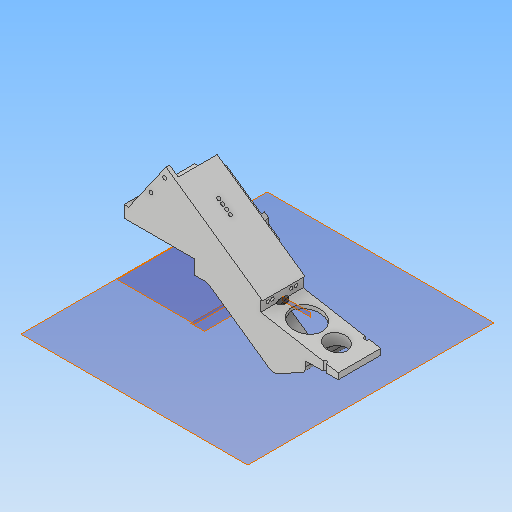
# Autodesk Inventor part: cellSTORM_inverted_opticsmodule_v0
Saved by Autodesk Inventor 2019.4 (Build 234330000, 330)
## iProperties
Created: 2020-11-06
Part Number: cellSTORM_inverted_opticsmodule_v0
Material: Generic
Document SubType Name: Modeling
Designer: diederichbenedict
Density: 1 g/cm^3
Appearance: Default
Author: diederichbenedict
Autodesk Inventor part; units mm, degrees
ref_plane "Work Plane3" through (-115.9521, -96.7438, -58.2763) normal (0, 0, -1) x (1, 0, 0)
sketch "Sketch1" plane through (-115.9521, -96.7438, -58.2763) normal (0, 0, -1) x (1, 0, 0)
  line L0 (-7, 0.25) -> (36, 0.25) construction
  line L1 (-7, 0.25) -> (-7, -8.45) construction
  line L2 (-7, -8.45) -> (-4, -8.45) construction
  line L3 (-4, -8.45) -> (-4, -14.75) construction
  line L4 (-1, -14.25) -> (-1, -7.5) construction
  line L5 (1, -17.25) -> (1, -14.75) construction
  line L6 (29, -17.25) -> (1, -17.25) construction
  line L7 (29, -14.75) -> (29, -17.25) construction
  line L8 (31, -14.75) -> (29, -14.75) construction
  line L9 (31, -17.25) -> (31, -14.75) construction
  line L10 (36, -17.25) -> (31, -17.25) construction
  line L11 (36, 0.25) -> (36, -17.25) construction
  line L12 (1, -7.5) -> (-1, -7.5) construction
  line L13 (1, -10) -> (1, -7.5) construction
  line L14 (29, -10) -> (1, -10) construction
  line L15 (29, -7.5) -> (29, -10) construction
  line L16 (31, -7.5) -> (29, -7.5) construction
  line L17 (31, -14.25) -> (31, -7.5) construction
  line L18 (-1, -14.25) -> (31, -14.25) construction
  line L19 (1, -0.25) -> (-1, -0.25) construction
  line L20 (1, -2.75) -> (1, -0.25) construction
  line L21 (29, -2.75) -> (1, -2.75) construction
  line L22 (29, -0.25) -> (29, -2.75) construction
  line L23 (31, -0.25) -> (29, -0.25) construction
  line L24 (31, -7) -> (31, -0.25) construction
  line L25 (-1, -7) -> (31, -7) construction
  line L26 (27.7903, 26.3233) -> (5.7037, 37.8208) construction
  line L27 (2.8269, 32.836) -> (5.3665, 37.7145) construction
  line L28 (25.357, 21.1075) -> (27.8966, 25.9861) construction
  line L29 (-43.6987, 4.97) -> (-31.4491, 13.5472) construction
  line L30 (-26.2161, -19.9978) -> (-13.9665, -11.4205) construction
  line L31 (-59.0209, -41.7593) -> (-53.082, -37.6009) construction
  line L32 (-75.3678, -18.4135) -> (-69.429, -14.2551) construction
  line L33 (-83.9784, -25.1198) -> (-79.8757, -30.9791) construction
  line L34 (31, 7.25) -> (31, 25.7798)
  line L35 (31, 25.7798) -> (3.201, 40.2511)
  line L36 (-100.2578, -32.1915) -> (-80.1961, -60.8425)
  line L37 (-80.1961, -60.8425) -> (-5.6575, -8.65)
  line L38 (-5.6575, -8.65) -> (-7.2, -8.65)
  line L39 (-7.2, -8.65) -> (-7.2, 0.45)
  line L40 (10.553, 27.4048) -> (-77.5642, -34.2955) construction
  line L41 (-7.2, 0.45) -> (31, 7.25)
  line L42 (-69.0481, -49.0348) -> (-79.0921, -56.3322) construction
  line L43 (-95.9265, -32.2901) -> (-85.6341, -25.3477) construction
  line L44 (-63.1835, 5.33) -> (-63.1835, -10.67) construction
  line L45 (-63.1835, -10.67) -> (-65.1835, -10.67) construction
  line L46 (-69.5218, -10.67) -> (-63.1835, -10.67)
  line L47 (-63.1835, -10.67) -> (-63.1835, -6.2318)
  line L48 (3.201, 40.2511) -> (-63.1835, -6.2318)
  line L49 (-69.5218, -10.67) -> (-100.2578, -32.1915)
  line L50 (1, -14.75) -> (-4, -14.75) projected
  line L51 (-1, -7) -> (-1, -0.25) projected
  point P0 (115.9521, -96.7438)
  point P1 (-1, -14.75)
  dimension "d1" = 1
  dimension "d3" = 0.2
  dimension "d4" = 0.2
  dimension "d6" = 0
  dimension "d7" = 0.2
  dimension "d8" = 7
  dimension "d9" = 3
  dimension "d92" = 0
  dimension "d114" = 95
  constraints: 34 end point, 3 perpendicular, 2 horizontal, 2 parallel, 1 point on line, 1 vertical, 15 other
  measures "d1" distance between parallel lines of L26 L35
  measures "d3" distance between parallel lines of L2 L38
  measures "d4" distance between parallel lines of L1 L39
  measures "d6" distance between parallel lines of L34 L24
  measures "d7" distance from line of L39.end L0
  measures "d8" distance from line of L0 L34.start
  measures "d9" distance from line of L36.end L42
  measures "d92" angle of L48 L37
  measures "d114" distance from line of L36 L0.start
extrude "Extrusion1" add sketch "Sketch1" against normal blind 3
ref_plane "Work Plane4" through (-106.9756, -82.4938, -91.2763) normal (0, 0, 1) x (1, 0, 0)
sketch "Sketch2" plane through (-115.9521, -96.7438, -58.2763) normal (0, 0, -1) x (-1, 0, 0)
  line L0 (-31, -25.7798) -> (-31, -7.25)
  line L1 (-3.201, -40.2511) -> (-31, -25.7798)
  line L2 (63.1835, 6.2318) -> (-3.201, -40.2511)
  line L3 (80.1961, 60.8425) -> (100.2578, 32.1915)
  line L4 (5.6575, 8.65) -> (80.1961, 60.8425)
  line L5 (7.2, 8.65) -> (5.6575, 8.65)
  line L6 (7.2, -0.45) -> (7.2, 8.65)
  line L7 (-31, -7.25) -> (7.2, -0.45)
  line L8 (59.0209, 41.7593) -> (53.082, 37.6009) construction
  line L9 (75.3678, 18.4135) -> (69.429, 14.2551)
  line L10 (-3.2205, -36.8588) -> (-28, -23.9593)
  line L11 (-28, -23.9593) -> (-28, -9.7631)
  line L12 (-28, -9.7631) -> (10.2, -2.9631)
  line L13 (10.2, -2.9631) -> (10.2, 11.65) construction
  line L14 (71.0992, 15.4246) -> (54.7523, 38.7704)
  line L15 (59.0209, 41.7593) -> (53.082, 37.6009)
  line L16 (65.1603, 11.2662) -> (48.8134, 34.612) construction
  line L17 (75.3678, 18.4135) -> (69.429, 14.2551)
  line L18 (46.6751, 33.3589) -> (61.0457, 12.8355)
  line L19 (82.2228, 22.9692) -> (75.8066, 18.4766)
  line L20 (10.2, 7.8187) -> (46.6751, 33.3589)
  line L21 (10.2, 7.8187) -> (26.7764, -15.8547)
  line L22 (10.2, -2.9631) -> (21.7105, -19.4019)
  line L23 (80.1961, 60.8425) -> (100.2578, 32.1915)
  line L24 (100.2578, 32.1915) -> (-3.201, -40.2511)
  line L25 (63.1835, 10.67) -> (63.1835, 6.2318)
  line L26 (69.5218, 10.67) -> (63.1835, 10.67)
  line L27 (100.2578, 32.1915) -> (69.5218, 10.67)
  line L28 (60.1835, 7.5372) -> (60.1835, 12.2317)
  line L29 (60.1835, 12.2317) -> (61.0457, 12.8355)
  line L30 (63.1835, 10.67) -> (63.1835, 6.2318)
  line L31 (60.1835, 7.5372) -> (-3.2205, -36.8588)
  line L32 (63.1835, 6.2318) -> (-3.201, -40.2511)
  line L33 (63.1835, 10.67) -> (63.1835, 6.2318)
  line L34 (63.1835, 6.2318) -> (63.1835, 10.67)
  line L35 (100.2578, 32.1915) -> (69.5218, 10.67)
  line L36 (63.1835, 10.67) -> (69.5218, 10.67)
  line L37 (69.5218, 10.67) -> (100.2578, 32.1915)
  line L38 (-28, -19.2299) -> (0.6537, -34.146)
  line L39 (75.3678, 18.4135) -> (59.0209, 41.7593) construction
  line L40 (59.0209, 41.7593) -> (53.082, 37.6009) construction
  line L41 (69.429, 14.2551) -> (53.082, 37.6009) construction
  line L42 (75.3678, 18.4135) -> (69.429, 14.2551) construction
  line L43 (75.3678, 18.4135) -> (59.0209, 41.7593) construction
  line L44 (59.0209, 41.7593) -> (53.082, 37.6009) construction
  line L45 (69.429, 14.2551) -> (53.082, 37.6009) construction
  line L46 (75.3678, 18.4135) -> (69.429, 14.2551) construction
  line L47 (75.3678, 18.4135) -> (59.0209, 41.7593) construction
  line L48 (59.0209, 41.7593) -> (53.082, 37.6009) construction
  line L49 (69.429, 14.2551) -> (53.082, 37.6009) construction
  line L50 (75.3678, 18.4135) -> (69.429, 14.2551) construction
  line L51 (69.429, 14.2551) -> (53.082, 37.6009) construction
  line L52 (75.3678, 18.4135) -> (69.429, 14.2551) construction
  line L53 (49.2033, 35.1291) -> (79.6237, 56.4297)
  line L54 (79.6237, 56.4297) -> (96.2, 32.7562)
  line L55 (96.2, 32.7562) -> (66.1366, 11.7056)
  line L56 (49.2033, 35.1291) -> (66.1366, 11.7056)
  line L57 (65.2751, 11.1023) -> (65.1603, 11.2662)
  line L58 (63.1835, 14.0894) -> (63.0694, 14.2524)
  line L59 (48.8134, 34.612) -> (48.6987, 34.7758)
  point P0 (-115.9521, 96.7438)
extrude "Extrusion2" add sketch "Sketch2" along normal up to surface (33 mm away) contours L0 L7 L6 L5 L4 L3 L24 L26 L25 L2 L1
sketch "Sketch3" plane through (-112.7316, -133.6026, -58.2763) normal (-0.4617486, 0.8870108, 0) x (0.8870108, 0.4617486, 0)
  circle A0 centre (14.2084, 15) radius 12.7 projected
  line L0 (0, 33) -> (27.936, 33) projected
  line L1 (0, 0) -> (0, 33) projected
  line L2 (27.936, 0) -> (0, 0) projected
  line L3 (27.936, 0) -> (27.936, 33) projected
  circle A1 centre (14.2084, 15) radius 13.2
  point P0 (161.685, -58.2763)
  dimension "d15" = 0.5
  constraints: 1 centre point
  measures "d15" radial gap between concentric circles of A0 A1
ref_plane "Work Plane5" through (-110.6706, -134.7844, -86.2023) normal (0.4617486, -0.8870108, 0) x (0.8863364, 0.4613975, -0.0389899)
extrude "Extrusion3" cut sketch "Sketch3" against normal blind 2.2 contours A0 | A1
sketch "Sketch4" plane through (-99.1128, -128.9933, -73.2763) normal (-0.4617486, 0.8870108, 0) x (0.8870108, 0.4617486, 0)
  circle A0 centre (0, 0) radius 13.2 projected
  circle A1 centre (0, 0) radius 8.2
  point P0 (147.4766, -73.2763)
  dimension "d18" = 5
  constraints: 1 centre point
  measures "d18" radial gap between concentric circles of A0 A1
extrude "Extrusion4" cut sketch "Sketch4" against normal blind 3 contours A1
ref_plane "Work Plane6" through (-115.6592, -109.4938, -86.9599) normal (0, 1, 0) x (0.2856174, 0, 0.9583437)
sketch "Sketch5" plane through (-128.1477, 0, -58.2763) normal (0, 1, 0) x (1, 0, 0)
  circle A0 centre (26.1721, 15) radius 12.15 projected
  circle A1 centre (26.1721, 15) radius 13
  point P0 (128.1477, -58.2763)
  point P1 (24.1765, 18)
  dimension "d145" = 26
  constraints: 1 centre point, 1 coincident
  measures "d145" diameter of A1
extrude "Extrusion5" cut sketch "Sketch5" against normal up to surface (109.4938 mm away) contours A0 | A1
sketch "Sketch6" plane through (-216.2099, -64.5523, -91.2763) normal (-0.819152, 0.5735764, 0) x (0, 0, 1)
  circle A0 centre (18, 17.24) radius 12.3
  circle A1 centre (18, 17.24) radius 14.6
  point P0 (91.2763, 176.891)
  dimension "d113" = 29.2
  constraints: 2 centre point, 2 other
  measures "d113" diameter of A1
extrude "Extrusion6" cut sketch "Sketch6" against normal up to surface (3 mm away) contours A0 | A1
sketch "Sketch10" plane through (-84.9521, -122.5236, -91.2763) normal (0, 0, -1) x (-1, 0, 0)
  line L0 (38.2, 25.3298) -> (0, 18.5298) construction
  line L1 (0, 18.5298) -> (0, 0) construction
  line L2 (0, 0) -> (27.799, -14.4713) construction
  line L3 (27.799, -14.4713) -> (94.1835, 32.0116) construction
  line L4 (131.2578, 57.9713) -> (111.1961, 86.6223) construction
  line L5 (111.1961, 86.6223) -> (36.6575, 34.4298) construction
  line L6 (36.6575, 34.4298) -> (38.2, 34.4298) construction
  line L7 (38.2, 34.4298) -> (38.2, 25.3298) construction
  line L8 (3, 1.8204) -> (3, 16.0167) construction
  line L9 (3, 16.0167) -> (41.2, 22.8167) construction
  line L10 (41.2, 22.8167) -> (52.7105, 6.3779) construction
  line L11 (27.7795, -11.079) -> (3, 1.8204) construction
  line L12 (96.1835, 36.4498) -> (152.1835, 36.4498) construction
  line L13 (94.1835, 20.4498) -> (94.1835, 36.4498) construction
  line L14 (154.1835, 20.4498) -> (154.1835, 36.4498) construction
  line L15 (100.5218, 36.4498) -> (154.1835, 36.4498) construction
  line L16 (100.5218, 36.4498) -> (154.1835, 36.4498) construction
  line L17 (131.2578, 57.9713) -> (27.799, -14.4713) construction
  line L18 (154.1835, 46.4498) -> (154.1835, 36.4498)
  line L19 (111.1961, 86.6223) -> (131.2578, 57.9713) construction
  line L20 (131.2578, 57.9713) -> (100.5218, 36.4498) construction
  line L21 (94.1835, 32.0116) -> (94.1835, 24.4498) construction
  line L22 (94.1835, 24.4498) -> (83.3841, 24.4498)
  line L23 (94.1835, 32.0116) -> (83.3841, 24.4498) construction
  line L24 (154.1835, 36.4498) -> (100.5218, 36.4498)
  line L25 (131.2578, 57.9713) -> (100.5218, 36.4498)
  line L26 (83.3841, 24.4498) -> (94.1835, 32.0116)
  line L27 (94.1835, 24.4498) -> (94.1835, 32.0116)
  line L28 (94.1835, 36.4498) -> (100.5218, 36.4498) projected
  line L29 (100.5218, 36.4498) -> (131.2578, 57.9713) projected
  line L30 (94.1835, 32.0116) -> (94.1835, 36.4498) projected
  line L31 (91.1835, 33.317) -> (57.7764, 9.925) projected
  line L32 (52.7105, 6.3779) -> (27.7795, -11.079) projected
  line L33 (57.7764, 9.925) -> (41.2, 33.5985) projected
  line L34 (41.2, 33.5985) -> (77.6751, 59.1387) projected
  line L35 (77.6751, 59.1387) -> (92.0457, 38.6153) projected
  line L36 (92.0457, 38.6153) -> (91.1835, 38.0115) projected
  line L37 (91.1835, 38.0115) -> (91.1835, 33.317) projected
  line L38 (83.3841, 24.4498) -> (81.7838, 26.7352)
  line L39 (127.2, 58.536) -> (97.1366, 37.4854) construction
  line L40 (57.7764, 9.925) -> (91.1835, 33.317) projected
  line L41 (81.7838, 26.7352) -> (91.1835, 33.317)
  line L42 (91.1835, 33.317) -> (91.1835, 38.0115) projected
  line L43 (91.1835, 33.317) -> (91.1835, 38.0115)
  line L44 (91.1835, 38.0115) -> (92.0457, 38.6153) construction
  line L45 (92.0457, 38.6153) -> (94.9309, 40.6355)
  line L46 (94.9309, 40.6355) -> (97.1366, 37.4854) construction
  line L47 (97.1366, 37.4854) -> (127.2, 58.536) construction
  line L48 (94.9309, 40.6355) -> (97.1366, 37.4854)
  line L49 (97.1366, 37.4854) -> (127.2, 58.536)
  line L50 (127.2, 58.536) -> (130.8624, 58.536)
  line L51 (100.5218, 36.4498) -> (131.2578, 57.9713) projected
  line L52 (130.8624, 58.536) -> (131.2578, 57.9713)
  line L53 (57.7764, 9.925) -> (91.1835, 33.317) projected
  line L54 (81.7838, 26.7352) -> (91.1835, 33.317)
  line L55 (91.1835, 33.317) -> (91.1835, 38.0115)
  line L56 (91.1835, 38.0115) -> (94.9309, 40.6355)
  line L57 (94.9309, 40.6355) -> (97.1366, 37.4854)
  line L58 (154.1835, 46.4498) -> (114.8033, 46.4498)
  line L59 (131.2578, 57.9713) -> (100.5218, 36.4498) projected
  point P0 (-84.9521, 122.5236)
  dimension "d38" = 12
  dimension "d149" = 10
  constraints: 50 end point, 13 point on line, 11 collinear, 7 perpendicular, 2 horizontal, 2 vertical, 1 parallel
  measures "d38" distance between parallel lines of L12 L22
  measures "d149" distance between parallel lines of L58 L12
ref_plane "Work Plane7" through (-237.1356, -102.0738, -103.2763) normal (0, 0, -1) x (0, 1, 0)
extrude "Extrusion10" add sketch "Sketch10" against normal blind 36 and the other way blind 24 contours L18 L24 L25 L58 | L27 L22 L26
sketch "Sketch11" plane through (-84.9521, -122.5236, -91.2763) normal (0, 0, -1) x (-1, 0, 0)
  line L0 (57.7764, 9.925) -> (91.1835, 33.317) projected
  line L1 (58.8799, 51.3735) -> (38, 37.4298) projected
  circle A0 centre (58.4518, 12.1681) radius 1.45
  line L2 (41.7774, 33.4536) -> (57.8377, 10.5172) projected
  line L3 (52.7105, 6.3779) -> (27.7795, -11.079) projected
  arc A1 (61.4816, 12.5195) -> (55.7249, 13.5345) centre (58.4518, 12.1681) ccw
  line L4 (91.1835, 33.317) -> (57.7764, 9.925) projected
  line L5 (38.2, 25.3298) -> (0, 18.5298) projected
  line L6 (0, 18.5298) -> (0, 0) projected
  line L7 (0, 0) -> (27.799, -14.4713) projected
  line L8 (27.799, -14.4713) -> (83.3841, 24.4498) projected
  line L9 (83.3841, 24.4498) -> (94.1835, 32.0116) projected
  line L10 (94.1835, 32.0116) -> (94.1835, 36.4498) projected
  line L11 (94.1835, 36.4498) -> (100.5218, 36.4498) projected
  line L12 (131.2578, 57.9713) -> (111.1961, 86.6223) projected
  line L13 (111.1961, 86.6223) -> (36.6575, 34.4298) projected
  line L14 (36.6575, 34.4298) -> (38.2, 34.4298) projected
  line L15 (38.2, 34.4298) -> (38.2, 25.3298) projected
  line L16 (3, 1.8204) -> (3, 16.0167) projected
  line L17 (3, 16.0167) -> (41.2, 22.8167) projected
  line L18 (41.2, 22.8167) -> (52.7105, 6.3779) projected
  line L19 (27.7795, -11.079) -> (3, 1.8204) projected
  circle A2 centre (50.6911, 6.734) radius 1.45
  line L20 (41.2, 22.8167) -> (52.7105, 6.3779) projected
  line L21 (52.7105, 6.3779) -> (27.7795, -11.079) projected
  line L22 (52.7105, 6.3779) -> (41.2, 22.8167) projected
  arc A3 (50.6911, 9.262) -> (49.8265, 4.3585) centre (50.6911, 6.734) ccw
  circle A4 centre (43.9558, 33.2951) radius 1.45
  circle A5 centre (43.9558, 33.2951) radius 3.503
  line L23 (41.2, 33.5985) -> (57.7764, 9.925) projected
  line L24 (41.2, 22.8167) -> (3, 16.0167) projected
  line L25 (3, 16.0167) -> (3, 1.8204) projected
  line L26 (3, 1.8204) -> (27.7795, -11.079) projected
  line L27 (52.7105, 6.3779) -> (41.2, 22.8167) projected
  line L28 (91.1835, 33.317) -> (91.1835, 38.0115) projected
  line L29 (91.1835, 38.0115) -> (92.0457, 38.6153) projected
  line L30 (92.0457, 38.6153) -> (77.6751, 59.1387) projected
  line L31 (77.6751, 59.1387) -> (41.2, 33.5985) projected
  line L32 (41.2, 33.5985) -> (57.7764, 9.925) projected
  line L33 (27.7795, -11.079) -> (52.7105, 6.3779) projected
  line L34 (52.7105, 6.3779) -> (27.7795, -11.079) projected
  line L35 (57.7764, 9.925) -> (41.2, 33.5985) projected
  line L36 (41.2, 33.5985) -> (77.6751, 59.1387) projected
  line L37 (77.6751, 59.1387) -> (92.0457, 38.6153) projected
  line L38 (92.0457, 38.6153) -> (91.1835, 38.0115) projected
  line L39 (91.1835, 38.0115) -> (91.1835, 33.317) projected
  line L40 (100.5218, 36.4498) -> (114.8033, 46.4498) projected
  line L41 (114.8033, 46.4498) -> (131.2578, 57.9713) projected
  point P0 (-84.9521, 122.5236)
  point P1 (61.747, 47.4364)
  point P2 (77.9448, 24.3035)
  point P3 (77.8072, 24.5)
  point P4 (43.8644, 29.7933)
  point P5 (45.3538, 36.5071)
  point P6 (40.4594, 33.08)
  point P7 (40.5297, 32.5651)
  dimension "d44" = 2.9
  dimension "d47" = 2.9
  dimension "d96" = 2.9
  constraints: 8 point on circle, 6 centre point, 4 point on line, 4 tangent, 3 coincident, 2 other
  measures "d44" diameter of A0
  measures "d47" diameter of A2
  measures "d96" diameter of A4
extrude "Extrusion11" add sketch "Sketch11" against normal up to surface (36 mm away) contours A3 L18 A2 L3 | A2 L18 L3
fillet "Fillet1" radius 7 6 edges at (-112.7512, -136.9949, -73.2763) (-84.9521, -122.5236, -73.2763) (-168.3362, -98.0738, -73.2763) (-112.7316, -133.6026, -74.7763) (-87.9521, -120.7032, -74.7763) (-87.9521, -106.5069, -74.7763)
sketch "Sketch13" plane through (-123.1521, -88.0938, -55.2763) normal (1, 0, 0) x (0, 0, -1)
  circle A0 centre (10, -4.4426) radius 1.45 projected
  circle A1 centre (26, -4.4426) radius 1.45 projected
  circle A2 centre (30, -4.4426) radius 1.45 projected
  circle A3 centre (6, -4.4426) radius 1.45 projected
  point P0 (-55.2763, 88.0938)
extrude "Extrusion13" cut sketch "Sketch13" against normal blind 25
sketch "Sketch16" plane through (-163.179, -96.2524, -91.2763) normal (0, 0, -1) x (-1, 0, 0)
  line L0 (53.0309, 31.7002) -> (32.9692, 60.3512) projected
  line L1 (32.9692, 60.3512) -> (-41.5694, 8.1586) projected
  line L2 (-78.2269, -7.7414) -> (-40.0269, -0.9414) projected
  line L3 (-78.2269, -7.7414) -> (-105.7935, -12.6485)
  line L4 (-105.2267, -17.7414) -> (-97.798, -17.7414) projected
  line L5 (-105.7935, -12.6485) -> (-105.7935, -17.7414)
  line L6 (-105.7935, -17.7414) -> (-78.2269, -17.7414)
  line L7 (-78.2269, -22.0234) -> (-78.2269, -7.7414) projected
  line L8 (-78.2269, -7.7414) -> (-78.2269, -17.7414)
  line L9 (-41.5694, 8.1586) -> (-40.0269, 8.1586) projected
  line L10 (-40.0269, 8.1586) -> (-40.0269, -0.9414) projected
  line L11 (-40.0269, -0.9414) -> (-78.2269, -7.7414) projected
  line L12 (-78.2269, -7.7414) -> (-78.2269, -22.0234) projected
  arc A0 (-78.2269, -22.0234) -> (-74.4591, -28.2325) centre (-71.2269, -22.0234) ccw projected
  line L13 (-74.4591, -28.2325) -> (-54.1956, -38.781) projected
  arc A1 (-54.1956, -38.781) -> (-46.9483, -38.306) centre (-50.9634, -32.572) ccw projected
  line L14 (-46.9483, -38.306) -> (3.3492, -3.0873) projected
  arc A2 (7.3643, -1.8214) -> (3.3492, -3.0873) centre (7.3643, -8.8214) ccw projected
  line L15 (5.1572, -1.8214) -> (7.3643, -1.8214) projected
  line L16 (5.1572, -1.8214) -> (15.9566, 5.7405) projected
  line L17 (15.9566, 5.7405) -> (15.9566, 10.1786) projected
  line L18 (15.9566, 10.1786) -> (22.2949, 10.1786) projected
  line L19 (-20.4505, -16.3461) -> (-37.0269, 7.3274) projected
  line L20 (-37.0269, 7.3274) -> (-0.5518, 32.8675) projected
  line L21 (-0.5518, 32.8675) -> (13.8188, 12.3441) projected
  line L22 (13.8188, 12.3441) -> (12.9566, 11.7403) projected
  line L23 (12.9566, 11.7403) -> (12.9566, 7.0458) projected
  line L24 (12.9566, 7.0458) -> (-20.4505, -16.3461) projected
  circle A3 centre (-27.5358, -19.5372) radius 1.45 projected
  arc A4 (-27.5358, -17.0092) -> (-28.4005, -21.9127) centre (-27.5358, -19.5372) ccw projected
  line L25 (-28.4005, -21.9127) -> (-46.9679, -34.9137) projected
  arc A5 (-54.2151, -35.3887) -> (-46.9679, -34.9137) centre (-50.9829, -29.1797) ccw projected
  line L26 (-54.2151, -35.3887) -> (-71.4591, -26.4121) projected
  arc A6 (-75.2269, -20.203) -> (-71.4591, -26.4121) centre (-68.2269, -20.203) ccw projected
  line L27 (-75.2269, -20.203) -> (-75.2269, -16.1185) projected
  arc A7 (-69.4537, -9.2268) -> (-75.2269, -16.1185) centre (-68.2269, -16.1185) ccw projected
  line L28 (-69.4537, -9.2268) -> (-37.0269, -3.4545) projected
  line L29 (-37.0269, -3.4545) -> (-27.5358, -17.0092) projected
  line L30 (22.2949, 10.1786) -> (36.5764, 20.1786) projected
  line L31 (36.5764, 20.1786) -> (53.0309, 31.7002) projected
  point P0 (-163.179, 96.2524)
  point P1 (-45.8001, -1.9691)
  dimension "d69" = 28
  constraints: 8 end point, 1 collinear, 1 point on line, 1 vertical
  measures "d69" distance of L2.start L3.end
extrude "Extrusion16" add sketch "Sketch16" against normal up to surface (36 mm away) contours L7 L6 L4 L5 L3
sketch "Sketch17" plane through (-84.9521, -113.9938, -91.2763) normal (0, -1, 0) x (1, 0, 0)
  arc A0 (8.0711, 22.55) -> (8.0711, 13.45) centre (8.0711, 18) ccw projected
  circle A1 centre (16.0711, 0.5) radius 2.1 projected
  arc A2 (16.0711, 37.6) -> (16.0711, 33.4) centre (16.0711, 35.5) ccw projected
  circle A3 centre (16.0711, 0.5) radius 1.7427
  circle A4 centre (16.0711, 35.5) radius 1.45
  circle A5 centre (8.0711, 18) radius 9
  point P0 (84.9521, 91.2763)
  dimension "d72" = 2.9
  dimension "d73" = 18
  constraints: 3 centre point, 3 coincident
  measures "d72" diameter of A4
  measures "d73" diameter of A5
extrude "Extrusion17" cut sketch "Sketch17" against normal through all contours A3 | A4 | A5
sketch "Sketch19" plane through (-84.9521, -122.5236, -115.2763) normal (0, 0, -1) x (-1, 0, 0)
  line L0 (31.259, -8.6426) -> (49.8265, 4.3585) projected
  line L1 (-14.4017, 15.9661) -> (-14.4017, 8.5298) projected
  line L2 (-14.4017, 8.5298) -> (0, 8.5298) projected
  line L3 (0, 8.5298) -> (0, 4.2477) projected
  arc A0 (0, 4.2477) -> (3.7678, -1.9614) centre (7, 4.2477) ccw projected
  line L4 (3.7678, -1.9614) -> (24.0313, -12.5099) projected
  arc A1 (24.0313, -12.5099) -> (31.2786, -12.0349) centre (27.2635, -6.3008) ccw projected
  line L5 (31.2786, -12.0349) -> (81.5761, 23.1839) projected
  arc A2 (85.5912, 24.4498) -> (81.5761, 23.1839) centre (85.5912, 17.4498) ccw projected
  line L6 (83.3841, 24.4498) -> (85.5912, 24.4498) projected
  line L7 (83.3841, 24.4498) -> (94.1835, 32.0116) projected
  line L8 (94.1835, 32.0116) -> (94.1835, 36.4498) projected
  line L9 (94.1835, 36.4498) -> (100.5218, 36.4498) projected
  line L10 (131.2578, 57.9713) -> (111.1961, 86.6223) projected
  line L11 (111.1961, 86.6223) -> (36.6575, 34.4298) projected
  line L12 (36.6575, 34.4298) -> (38.2, 34.4298) projected
  line L13 (38.2, 34.4298) -> (38.2, 25.3298) projected
  line L14 (38.2, 25.3298) -> (-14.4017, 15.9661) projected
  circle A3 centre (50.6911, 6.734) radius 1.45 projected
  line L15 (77.6751, 59.1387) -> (92.0457, 38.6153) projected
  line L16 (92.0457, 38.6153) -> (91.1835, 38.0115) projected
  line L17 (91.1835, 38.0115) -> (91.1835, 33.317) projected
  line L18 (91.1835, 33.317) -> (57.7764, 9.925) projected
  line L19 (57.7764, 9.925) -> (41.2, 33.5985) projected
  line L20 (41.2, 33.5985) -> (77.6751, 59.1387) projected
  line L21 (49.8265, 4.3585) -> (31.259, -8.6426) projected
  arc A4 (24.0118, -9.1176) -> (31.259, -8.6426) centre (27.244, -2.9085) ccw projected
  line L22 (24.0118, -9.1176) -> (6.7678, -0.1409) projected
  arc A5 (3, 6.0681) -> (6.7678, -0.1409) centre (10, 6.0681) ccw projected
  line L23 (3, 6.0681) -> (3, 10.1527) projected
  arc A6 (8.7732, 17.0444) -> (3, 10.1527) centre (10, 10.1527) ccw projected
  line L24 (8.7732, 17.0444) -> (41.2, 22.8167) projected
  line L25 (41.2, 22.8167) -> (50.6911, 9.262) projected
  arc A7 (50.6911, 9.262) -> (49.8265, 4.3585) centre (50.6911, 6.734) ccw projected
  line L26 (57.7764, 9.925) -> (91.1835, 33.317) projected
  line L27 (83.3841, 24.4498) -> (94.1835, 32.0116) projected
  line L28 (83.3841, 24.4498) -> (81.7838, 26.7352)
  line L29 (81.7838, 26.7352) -> (91.1835, 33.317)
  line L30 (91.1835, 38.0115) -> (92.0457, 38.6153) projected
  line L31 (91.1835, 33.317) -> (91.1835, 38.0115)
  line L32 (91.1835, 33.317) -> (91.1835, 38.0115) projected
  line L33 (91.1835, 38.0115) -> (94.9309, 40.6355)
  line L34 (94.9309, 40.6355) -> (97.1366, 37.4854)
  line L35 (97.1366, 37.4854) -> (127.2, 58.536) projected
  line L36 (97.1366, 37.4854) -> (127.2, 58.536)
  line L37 (127.2, 58.536) -> (130.8624, 58.536)
  line L38 (111.1961, 86.6223) -> (131.2578, 57.9713) projected
  line L39 (130.8624, 58.536) -> (127.162, 55.1034)
  line L40 (127.162, 55.1034) -> (100.5218, 36.4498)
  line L41 (100.5218, 36.4498) -> (94.1835, 36.4498)
  line L42 (94.1835, 36.4498) -> (94.1835, 32.0116)
  line L43 (98.2792, 34.8795) -> (83.3841, 24.4498)
  line L44 (100.5218, 36.4498) -> (114.8033, 46.4498) projected
  line L45 (114.8033, 46.4498) -> (131.2578, 57.9713) projected
  point P0 (-84.9521, 122.5236)
  point P1 (107.1198, 75.0095)
  point P2 (94.1835, 24.4498)
  constraints: 24 end point, 4 point on line, 3 perpendicular, 1 collinear, 1 horizontal, 1 parallel, 1 vertical, 2 other
extrude "Extrusion19" add sketch "Sketch19" against normal up to surface (24 mm away) contours L39 L40 L9 L8 L7 L28 L18 L17 L16 L33 L34 L35 L37 | L10 L45 L39
ref_plane "Work Plane9" through (-239.1356, -131.0738, -115.2763) normal (0, -1, 0) x (1, 0, 0)
ref_plane "Work Plane10" through (-239.1356, -131.0738, -115.2763) normal (0, -1, 0) x (1, 0, 0)
sketch "Sketch23" plane through (-115.9521, -96.7438, -55.2763) normal (0, 0, 1) x (1, 0, 0)
  line L0 (-80.1961, 60.8425) -> (-100.2578, 32.1915) projected
  line L1 (-99.8624, 32.7562) -> (-80.1961, 60.8425) projected
  line L2 (-80.1961, 60.8425) -> (-87.5685, 66.0047)
  line L3 (-87.5685, 66.0047) -> (-119.3122, 20.67)
  line L4 (-119.3122, 20.67) -> (-119.3122, 20.67)
  line L5 (-123.1835, 20.67) -> (-83.8033, 20.67) projected
  line L6 (-119.3122, 20.67) -> (-83.8033, 20.67)
  line L7 (-83.8033, 20.67) -> (-100.2578, 32.1915)
  line L8 (-80.1961, 60.8425) -> (-100.2578, 32.1915)
  line L9 (-100.2578, 32.1915) -> (-83.8033, 20.67)
  line L10 (-83.8033, 20.67) -> (-119.3122, 20.67)
  line L11 (-83.8033, 20.67) -> (-123.1835, 20.67) projected
  circle A0 centre (-100.2756, 41.0424) radius 1.6 projected
  circle A1 centre (-88.8041, 57.4255) radius 1.6 projected
  point P0 (115.9521, 96.7438)
  point P1 (-96.162, 29.3237)
  dimension "d146" = 9
  constraints: 16 end point, 3 collinear, 2 perpendicular, 2 point on line, 1 horizontal, 1 vertical, 1 other
extrude "Extrusion22" add sketch "Sketch23" against normal blind 3
sketch "Sketch24" plane through (-123.1521, -97.1938, -91.2763) normal (0, 0, -1) x (-1, 0, 0)
  line L0 (52.8428, 8.1328) -> (36.4959, 31.4786) construction
  line L1 (36.4959, 31.4786) -> (30.557, 27.3202) construction
  line L2 (46.9039, 3.9744) -> (30.557, 27.3202) construction
  line L3 (52.8428, 8.1328) -> (46.9039, 3.9744) construction
  line L4 (42.6395, 35.7805) -> (58.9864, 12.4346) construction
  line L5 (58.9864, 12.4346) -> (64.9253, 16.5931) construction
  line L6 (48.5783, 39.9389) -> (64.9253, 16.5931) construction
  line L7 (42.6395, 35.7805) -> (48.5783, 39.9389) construction
  circle A0 centre (12.4911, -18.5958) radius 1.45 construction
  line L8 (89, 33.2062) -> (92.6624, 33.2062) construction
  line L9 (92.6624, 33.2062) -> (72.9961, 61.2925) construction
  line L10 (72.9961, 61.2925) -> (-1.5425, 9.1) construction
  line L11 (-1.5425, 9.1) -> (0, 9.1) construction
  line L12 (0, 9.1) -> (0, 0) construction
  line L13 (0, 0) -> (-52.6017, -9.3636) construction
  line L14 (-52.6017, -9.3636) -> (-52.6017, -16.8) construction
  line L15 (-52.6017, -16.8) -> (-38.2, -16.8) construction
  line L16 (-38.2, -16.8) -> (-38.2, -21.0821) construction
  arc A1 (-38.2, -21.0821) -> (-34.4322, -27.2912) centre (-31.2, -21.0821) ccw construction
  line L17 (-34.4322, -27.2912) -> (-14.1687, -37.8397) construction
  arc A2 (-14.1687, -37.8397) -> (-6.9214, -37.3647) centre (-10.9365, -31.6306) ccw construction
  line L18 (-6.9214, -37.3647) -> (43.3761, -2.1459) construction
  arc A3 (47.3912, -0.88) -> (43.3761, -2.1459) centre (47.3912, -7.88) ccw construction
  line L19 (45.1841, -0.88) -> (47.3912, -0.88) construction
  line L20 (45.1841, -0.88) -> (43.5838, 1.4054) construction
  line L21 (43.5838, 1.4054) -> (19.5764, -15.4047) construction
  line L22 (19.5764, -15.4047) -> (3, 8.2687) construction
  line L23 (3, 8.2687) -> (39.4751, 33.8089) construction
  line L24 (39.4751, 33.8089) -> (53.8457, 13.2855) construction
  line L25 (53.8457, 13.2855) -> (56.6834, 15.2724) construction
  line L26 (56.6834, 15.2724) -> (42.0033, 35.5791) construction
  line L27 (42.0033, 35.5791) -> (72.4237, 56.8797) construction
  line L28 (72.4237, 56.8797) -> (89, 33.2062) construction
  line L29 (11.6265, -20.9713) -> (-6.941, -33.9724) construction
  arc A4 (-14.1882, -34.4474) -> (-6.941, -33.9724) centre (-10.956, -28.2383) ccw construction
  line L30 (-14.1882, -34.4474) -> (-31.4322, -25.4707) construction
  arc A5 (-35.2, -19.2616) -> (-31.4322, -25.4707) centre (-28.2, -19.2616) ccw construction
  line L31 (-35.2, -19.2616) -> (-35.2, -15.1771) construction
  arc A6 (-29.4268, -8.2854) -> (-35.2, -15.1771) centre (-28.2, -15.1771) ccw construction
  line L32 (-29.4268, -8.2854) -> (3, -2.5131) construction
  line L33 (3, -2.5131) -> (12.4911, -16.0678) construction
  arc A7 (12.4911, -16.0678) -> (11.6265, -20.9713) centre (12.4911, -18.5958) ccw construction
  line L34 (30.2785, 27.3693) -> (28.6402, 26.2222)
  line L35 (28.6402, 26.2222) -> (29.7873, 24.5839)
  line L36 (29.7873, 24.5839) -> (31.4256, 25.731)
  line L37 (31.4256, 25.731) -> (30.2785, 27.3693)
  line L38 (39.4751, 33.8089) -> (3, 8.2687) projected
  line L39 (36.545, 31.7572) -> (38.1833, 32.9043)
  line L40 (38.1833, 32.9043) -> (39.3304, 31.266)
  line L41 (39.3304, 31.266) -> (37.6921, 30.1189)
  line L42 (37.6921, 30.1189) -> (36.545, 31.7572)
  line L43 (19.5764, -15.4047) -> (52.9835, 7.9872) projected
  line L44 (46.8548, 3.6958) -> (45.2165, 2.5487)
  line L45 (45.2165, 2.5487) -> (44.0694, 4.187)
  line L46 (44.0694, 4.187) -> (45.7077, 5.3341)
  line L47 (45.7077, 5.3341) -> (46.8548, 3.6958)
  line L48 (52.9835, 7.9872) -> (52.9835, 12.6817) projected
  line L49 (52.9835, 8.2806) -> (51.9742, 9.722)
  line L50 (51.9742, 9.722) -> (52.9835, 10.4287)
  line L51 (52.9835, 8.2806) -> (52.9835, 10.4287)
  point P0 (-123.1521, 97.1938)
  dimension "d150" = 2
  dimension "d151" = 2
  dimension "d152" = 2
  dimension "d153" = 2
  dimension "d154" = 0.2
  dimension "d155" = 0.2
  dimension "d156" = 2
  dimension "d157" = 2
  constraints: 30 end point, 7 point on line, 6 parallel, 4 perpendicular, 1 collinear
  measures "d150" distance of L35.end L34.end
  measures "d151" distance between parallel lines of L35 L37
  measures "d152" distance of L39.end L40.end
  measures "d153" distance between parallel lines of L40 L42
  measures "d154" distance between parallel lines of L0 L42
  measures "d155" distance between parallel lines of L2 L37
  measures "d156" distance of L44.start L44.end
  measures "d157" distance of L44.end L45.end
extrude "Extrusion23" add sketch "Sketch24" against normal up to surface (33 mm away)
ref_plane "Work Plane11" through (-113.9278, -136.0738, -15.7746) normal (0, -1, 0) x (0, 0, -1)
ref_plane "Work Plane12" through (-179.1356, -132.0738, -115.2763) normal (0, -1, 0) x (1, 0, 0)
sketch "Sketch26" plane through (-179.1356, -132.0738, -115.2763) normal (0, -1, 0) x (1, 0, 0)
  circle A0 centre (102.2545, 42) radius 9 projected
  circle A1 centre (55.139, 42) radius 4.5
  point P0 (179.1356, 115.2763)
  dimension "d166" = 9
  constraints: 1 centre point
  measures "d166" diameter of A1
extrude "Extrusion25" add sketch "Sketch26" along normal blind 2 and the other way blind 9 contours A1
sketch "Sketch27" plane through (-123.9966, -134.0738, -73.2763) normal (0, -1, 0) x (1, 0, 0)
  circle A0 centre (0, 0) radius 4.5 projected
  point P0 (123.9966, 73.2763)
hole "Hole2" at (-123.9966, -134.0738, -73.2763) direction (0, 1, 0) diameter 2.9 depth 20 tip angle 118 counterbore diameter 7 counterbore depth 2.9
ref_plane "Work Plane13" through (-113.4411, -129.4624, -86.2023) normal (-0.4617486, 0.8870108, 0) x (0.0345845, 0.0180036, 0.9992396)
sketch "Sketch28" plane through (-126.1521, -99.7069, -58.2763) normal (0.819152, -0.5735764, 0) x (0, 0, -1)
  circle A0 centre (15, -5.618) radius 2.5 projected
  circle A1 centre (15, -5.618) radius 10.9635
  point P0 (-58.2763, 154.033)
  constraints: 1 centre point, 1 coincident
extrude "Extrusion26" cut sketch "Sketch28" along normal up to surface from surface at -90.9349 contours A0 | A1 surface through (-113.4411, -129.4624, -86.2023) normal (-0.4617486, 0.8870108, 0)
sketch "Sketch29" plane through (-121.6096, -88.0938, -55.2763) normal (0.5735764, 0.819152, 0) x (0.819152, -0.5735764, 0)
  line L0 (-90.9949, 36) -> (-90.9949, 3) projected
  line L1 (-99.9949, 3) -> (-90.9949, 3) projected
  line L2 (-99.9949, 0) -> (-99.9949, 3) projected
  line L3 (0, 0) -> (-99.9949, 0) projected
  line L4 (0, 36) -> (0, 0) projected
  line L5 (-90.9949, 36) -> (0, 36) projected
  circle A0 centre (-55.2427, 18) radius 1.45
  circle A1 centre (-59.2427, 18) radius 1.45
  circle A2 centre (-63.2427, 18) radius 1.45
  circle A3 centre (-67.2427, 18) radius 1.45
  point P0 (49.0882, -55.2763)
  dimension "d180" = 2.9
  dimension "d183" = 4
  constraints: 4 centre point, 1 horizontal, 6 other
  measures "d180" diameter of A0
  measures "d183" distance of A0.centre A1.centre
extrude "Extrusion27" cut sketch "Sketch29" against normal up to surface (3.2864 mm away) contours A0 | A1 | A2 | A3
sketch "Sketch30" plane through (-239.1356, -76.0738, -115.2763) normal (0, 1, 0) x (1, 0, 0)
  line L0 (3.8712, -57) -> (39.3801, -57) projected
  line L1 (39.3801, 0) -> (39.3801, -57) projected
  line L2 (0, 0) -> (39.3801, 0) projected
  line L3 (0, 0) -> (0, -60) projected
  line L4 (3.8712, -60) -> (0, -60) projected
  line L5 (3.8712, -60) -> (3.8712, -57) projected
  circle A0 centre (30, -5) radius 1.95 projected
  circle A1 centre (55, -5) radius 1.95 projected
  circle A2 centre (5, -5) radius 1.95 projected
  circle A3 centre (5, -30) radius 1.95 projected
  circle A4 centre (5, -55) radius 1.95 projected
  circle A5 centre (5, -30) radius 1.95 projected
  circle A6 centre (30, -55) radius 1.95 projected
  point P0 (239.1356, -115.2763)
  point P1 (18.8712, -57)
  point P2 (15, 0)
  point P3 (15, -60)
  point P4 (18.8712, -60)
  point P5 (20, -5)
  point P6 (20, -30)
  point P7 (20, -55)
  point P8 (20, -30)
  point P9 (40, -5)
  dimension "d192" = 15
  dimension "d204" = 15
  constraints: 1 horizontal, 8 other
  measures "d192" distance of L0.start point (18.871, -57)
  measures "d204" distance of point (40, -5) A1.centre
hole "Hole3" at (-234.1356, -76.0738, -60.2763) at (-234.1356, -76.0738, -85.2763) at (-234.1356, -76.0738, -110.2763) at (-219.1356, -76.0738, -110.2763) at (-219.1356, -76.0738, -85.2763) at (-219.1356, -76.0738, -60.2763) at (-199.1356, -76.0738, -110.2763) at (-184.1356, -76.0738, -110.2763) direction (0, -1, 0) diameter 2.9 end through all both
body "Solid1"
